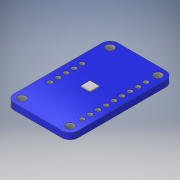
# Autodesk Inventor part: LSM9DS1
Saved by Autodesk Inventor 2019.4 (Build 234330000, 330)
## iProperties
Created: 2019-12-27
Part Number: LSM9DS1
Material: Generic
Document SubType Name: Modeling
Designer: Jorian Bruslind
Density: 1 g/cm^3
Appearance: Default
Author: Jorian Bruslind
Autodesk Inventor part; units mm, degrees
ref_plane "YZ Plane" through (0, 0, 0) normal (1, 0, 0) x (0, 1, 0)
ref_plane "XZ Plane" through (0, 0, 0) normal (0, 1, 0) x (-1, 0, 0)
ref_plane "XY Plane" through (0, 0, 0) normal (0, 0, 1) x (1, 0, 0)
sketch "Sketch1" plane through (0, 0, 0) normal (0, 1, 0) x (-1, 0, 0)
  line L0 (0, 0) -> (10.16, 0)
  line L1 (10.16, 0) -> (10.16, -13.97)
  line L2 (10.16, 0) -> (10.16, 13.97)
  line L3 (10.16, 0) -> (24.13, 0) construction
  line L4 (0, 0) -> (-10.16, 0)
  line L5 (0, 0) -> (10.16, 0) construction
  line L6 (-10.16, 0) -> (-10.16, -13.97)
  line L7 (-10.16, 0) -> (-10.16, 13.97)
  line L8 (-10.16, 13.97) -> (-7.62, 13.97)
  arc A0 (-7.62, 16.51) -> (-10.16, 13.97) centre (-7.62, 13.97) ccw
  line L9 (-7.62, 13.97) -> (-7.62, 16.51) construction
  line L10 (-7.62, 13.97) -> (-10.16, 13.97) construction
  line L11 (0, 0) -> (0, -1)
  line L12 (10.16, 13.97) -> (7.62, 13.97)
  line L13 (10.16, 13.97) -> (12.7, 13.97) construction
  arc A1 (10.16, 13.97) -> (7.62, 16.51) centre (7.62, 13.97) ccw
  line L14 (7.62, 13.97) -> (7.62, 16.51) construction
  line L15 (7.62, 13.97) -> (10.16, 13.97) construction
  line L16 (-7.62, 16.51) -> (7.62, 16.51)
  line L17 (10.16, -13.97) -> (7.62, -13.97)
  line L18 (10.16, -13.97) -> (12.7, -13.97) construction
  line L19 (-10.16, -13.97) -> (-7.62, -13.97)
  arc A2 (7.62, -16.51) -> (10.16, -13.97) centre (7.62, -13.97) ccw
  arc A3 (-10.16, -13.97) -> (-7.62, -16.51) centre (-7.62, -13.97) ccw
  line L20 (-7.62, -16.51) -> (7.62, -16.51)
  dimension "d0" = 10.16
  dimension "d1" = 13.97
  dimension "d2" = 13.97
  dimension "d3" = 90
  dimension "d4" = 10.16
  dimension "d5" = 180
  dimension "d6" = 13.97
  dimension "d7" = 13.97
  dimension "d8" = 2.54
  dimension "d9" = 90
  dimension "d11" = 1
  dimension "d12" = 2.54
  dimension "d13" = 180
  dimension "d14" = 90
  dimension "d15" = 2.54
  dimension "d16" = 180
  dimension "d17" = 2.54
  dimension "d18" = 15.24
  constraints: 42 end point, 11 horizontal, 8 point on circle, 4 centre point, 4 coincident, 4 equal length, 3 perpendicular, 2 vertical
  measures "d0" distance of L0.start L0.end
  measures "d1" distance of L0.end L1.end
  measures "d2" distance of L0.end L2.end
  measures "d3" angle of L3 L2
  measures "d4" distance of L0.start L4.end
  measures "d5" angle of L4 L5
  measures "d6" distance of L4.end L6.end
  measures "d7" distance of L4.end L7.end
  measures "d8" distance of L7.end L8.end
  measures "d9" angle of L9 L10
  measures "d11" distance of L0.start L11.end
  measures "d12" distance of L2.end L12.end
  measures "d13" angle of L12 L13
  measures "d14" angle of L15 L14
  measures "d15" distance of L1.end L17.end
  measures "d16" angle of L17 L18
  measures "d17" distance of L6.end L19.end
  measures "d18" distance of L20.start L20.end
extrude "Extrusion1" add sketch "Sketch1" along normal blind 2
sketch "Sketch2" plane through (0, 2, 0) normal (0, 1, 0) x (1, 0, 0)
  line L0 (0, 0) -> (7.62, 0)
  line L1 (0, 0) -> (-7.62, 0)
  circle A0 centre (7.62, 0) radius 0.75
  line L2 (0, 0) -> (0, 1)
  circle A1 centre (7.62, 2.54) radius 0.75
  circle A2 centre (7.62, 5.08) radius 0.75
  circle A3 centre (7.62, 7.62) radius 0.75
  circle A4 centre (7.62, 10.16) radius 0.75
  circle A5 centre (7.62, -2.54) radius 0.75
  circle A6 centre (7.62, 0) radius 0.75
  circle A7 centre (7.62, 2.54) radius 0.75
  circle A8 centre (7.62, 5.08) radius 0.75
  circle A9 centre (7.62, 7.62) radius 0.75
  circle A10 centre (7.62, -5.08) radius 0.75
  circle A11 centre (7.62, -2.54) radius 0.75
  circle A12 centre (7.62, 0) radius 0.75
  circle A13 centre (7.62, 2.54) radius 0.75
  circle A14 centre (7.62, 5.08) radius 0.75
  circle A15 centre (7.62, -7.62) radius 0.75
  circle A16 centre (7.62, -5.08) radius 0.75
  circle A17 centre (7.62, -2.54) radius 0.75
  circle A18 centre (7.62, 0) radius 0.75
  circle A19 centre (7.62, 2.54) radius 0.75
  circle A20 centre (7.62, -10.16) radius 0.75
  circle A21 centre (7.62, -7.62) radius 0.75
  circle A22 centre (7.62, -5.08) radius 0.75
  circle A23 centre (7.62, -2.54) radius 0.75
  circle A24 centre (7.62, 0) radius 0.75
  circle A25 centre (-7.62, 0) radius 0.75
  circle A26 centre (-7.62, 2.54) radius 0.75
  circle A27 centre (-7.62, 5.08) radius 0.75
  circle A28 centre (-7.62, -2.54) radius 0.75
  circle A29 centre (-7.62, 0) radius 0.75
  circle A30 centre (-7.62, 2.54) radius 0.75
  circle A31 centre (-7.62, -5.08) radius 0.75
  circle A32 centre (-7.62, -2.54) radius 0.75
  circle A33 centre (-7.62, 0) radius 0.75
  dimension "d21" = 7.62
  dimension "d22" = 7.62
  dimension "d23" = 1.5
  dimension "d24" = 1
  dimension "d27" = 2.54
  dimension "d30" = 2.54
  dimension "d33" = 1.5
  dimension "d36" = 2.54
  dimension "d39" = 2.54
  constraints: 34 centre point, 6 end point, 5 vertical, 2 coincident, 2 horizontal, 64 other
  measures "d21" distance of L0.start L0.end
  measures "d22" distance of L0.start L1.end
  measures "d23" diameter of A0
  measures "d24" distance of L0.start L2.end
  measures "d27" distance of A0.centre A1.centre
  measures "d30" distance of A0.centre A5.centre
  measures "d33" diameter of A25
  measures "d36" distance of A25.centre A26.centre
  measures "d39" distance of A25.centre A28.centre
extrude "Extrusion2" cut sketch "Sketch2" against normal blind 2
sketch "Sketch3" plane through (0, 2, 0) normal (0, 1, 0) x (1, 0, 0)
  line L0 (1.5, -1.5) -> (-1.5, -1.5)
  line L1 (-1.5, -1.5) -> (-1.5, 1.5)
  line L2 (-1.5, 1.5) -> (1.5, 1.5)
  line L3 (1.5, 1.5) -> (1.5, -1.5)
  line L4 (1.5, -1.5) -> (-1.5, 1.5) construction
  line L5 (-1.5, -1.5) -> (1.5, 1.5) construction
  point P0 (0, 0)
  dimension "d44" = 3
  dimension "d45" = 3
  constraints: 12 end point, 2 midpoint, 2 parallel, 1 horizontal, 1 perpendicular
  measures "d44" distance of L1.end L2.end
  measures "d45" distance of L0.end L1.end
extrude "Extrusion3" add sketch "Sketch3" along normal blind 0.25
sketch "Sketch4" plane through (0, 2, 0) normal (0, 1, 0) x (1, 0, 0)
  arc A0 (7.62, -16.51) -> (10.16, -13.97) centre (7.62, -13.97) ccw projected
  circle A1 centre (7.62, -13.97) radius 1.27
  line L0 (1.5, -1.5) -> (1.5, 1.5) projected
  line L1 (1.5, -1.5) -> (1.5, 1.5)
  line L2 (-1.5, 1.5) -> (-1.5, -1.5) projected
  line L3 (1.5, 1.5) -> (-1.5, 1.5)
  circle A2 centre (7.62, 13.97) radius 1.27
  circle A3 centre (-7.62, -13.97) radius 1.27
  circle A4 centre (-7.62, 13.97) radius 1.27
  point P0 (0, 0)
  dimension "d48" = 2.54
  dimension "d51" = 27.94
  dimension "d54" = 15.24
  constraints: 4 centre point, 4 end point, 1 coincident, 1 collinear, 1 horizontal, 1 perpendicular, 1 vertical, 6 other
  measures "d48" diameter of A1
  measures "d51" distance of A1.centre A2.centre
  measures "d54" distance of A1.centre A3.centre
extrude "Extrusion4" cut sketch "Sketch4" against normal blind 2
body "Solid1"
